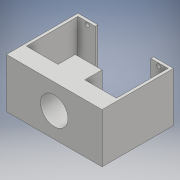
# Autodesk Inventor part: SoporteCuello
Saved by Autodesk Inventor 2017 SP1 (Build 210196100, 196)
## iProperties
Part Number: SoporteCuello
Material: Genérico
Document SubType Name: Modeling
Designer: Juan
Density: 1 g/cm^3
Appearance: Valor por defecto
Author: Juan
Autodesk Inventor part; units mm, degrees
sketch "Boceto1" plane through (0, 0, 0) normal (0, 1, 0) x (-1, 0, 0)
  line L0 (69.5, 36) -> (0, 36)
  line L1 (0, 36) -> (0, 0)
  line L2 (0, 0) -> (69.5, 0)
  line L3 (69.5, 0) -> (69.5, 36)
  dimension "d0" = 69.5
  dimension "d1" = 36
  constraints: 8 end point, 2 parallel, 1 coincident, 1 horizontal, 1 perpendicular
  measures "d0" distance of L2.end L1.end
  measures "d1" distance of L0.end L1.end
extrude "Extrusión1" add sketch "Boceto1" along normal blind 25
ref_plane "Plano de trabajo1" through (0, 25, 0) normal (0, 1, 0) x (1, 0, 0)
sketch "Boceto3" plane through (0, 25, 0) normal (0, 1, 0) x (1, 0, 0)
  line L0 (0, -36) -> (0, 0) projected
  line L1 (-69.5, -36) -> (0, -36) projected
  line L2 (0, 0) -> (-2, 0)
  line L3 (-2, 0) -> (-2, -36)
  line L4 (-2, -36) -> (0, -36)
  line L5 (0, -36) -> (0, 0)
  line L6 (0, 0) -> (-69.5, 0) projected
  line L7 (-69.5, 0) -> (-67.5, 0)
  line L8 (-67.5, 0) -> (-67.5, -36)
  line L9 (-67.5, -36) -> (-69.5, -36)
  line L10 (-69.5, -36) -> (-69.5, 0)
  dimension "d9" = 2
  dimension "d10" = 2
  constraints: 16 end point, 4 parallel, 2 horizontal, 2 perpendicular, 2 point on line
  measures "d9" distance of L4.end L3.end
  measures "d10" distance of L8.end L9.end
extrude "Extrusión3" add sketch "Boceto3" along normal blind 27 contours L1 L3 L2 L0 | L1 L10 L6 L8
ref_plane "Plano de trabajo2" through (-67.5, 25, 36) normal (1, 0, 0) x (0, 0, -1)
ref_plane "Plano de trabajo3" through (-2, 25, 0) normal (-1, 0, 0) x (0, 0, 1)
sketch "Boceto5" plane through (-67.5, 25, 36) normal (1, 0, 0) x (0, 0, -1)
  line L0 (0, 0) -> (0, 27) projected
  line L1 (36, 0) -> (36, 27) projected
  line L2 (0, 27) -> (36, 27)
  line L3 (36, 27) -> (36, 25)
  line L4 (36, 25) -> (0, 25)
  line L5 (0, 25) -> (0, 27)
  point P0 (36, -25)
  dimension "d15" = 2
  constraints: 8 end point, 2 parallel, 1 horizontal, 1 perpendicular, 1 point on line
  measures "d15" distance of L2.end L3.end
sketch "Boceto6" plane through (-2, 25, 0) normal (-1, 0, 0) x (0, 0, 1)
  line L0 (0, 0) -> (0, 27) projected
  line L1 (36, 0) -> (36, 27) projected
  line L2 (0, 27) -> (36, 27)
  line L3 (36, 27) -> (36, 25)
  line L4 (36, 25) -> (0, 25)
  line L5 (0, 25) -> (0, 27)
  point P0 (0, -25)
  dimension "d16" = 2
  constraints: 8 end point, 2 parallel, 1 horizontal, 1 perpendicular, 1 point on line
  measures "d16" distance of L2.end L3.end
extrude "Extrusión4" add sketch "Boceto5" along normal blind 12.5
extrude "Extrusión5" add sketch "Boceto6" along normal blind 12.5
ref_plane "Plano de trabajo4" through (0, 52, 0) normal (0, 1, 0) x (1, 0, 0)
ref_plane "Plano de trabajo5" through (0, 52, 0) normal (0, 1, 0) x (1, 0, 0)
sketch "Boceto7" plane through (0, 52, 0) normal (0, 1, 0) x (1, 0, 0)
  line L0 (0, -36) -> (0, 0) construction
  line L1 (0, -36) -> (-8.75, -36) construction
  line L2 (0, -36) -> (-14.5, -36) construction
  line L3 (-8.75, -36) -> (-8.75, -34) construction
  line L4 (0, 0) -> (-8.75, 0) construction
  line L5 (0, 0) -> (-14.5, 0) construction
  line L6 (-8.75, 0) -> (-8.75, -2) construction
  line L7 (-69.5, -36) -> (0, -36) construction
  line L8 (-69.5, -36) -> (-60.75, -36) construction
  line L9 (-60.75, -36) -> (-60.75, -34) construction
  line L10 (-69.5, 0) -> (-60.75, 0) construction
  line L11 (-60.75, 0) -> (-60.75, -2) construction
  dimension "d23" = 8.75
  dimension "d24" = 2
  dimension "d25" = 8.75
  dimension "d26" = 2
  dimension "d27" = 8.75
  dimension "d28" = 2
  dimension "d29" = 8.75
  constraints: 16 end point, 3 point on line, 2 perpendicular, 2 vertical
  measures "d23" distance of L0.start L1.end
  measures "d24" distance of L1.end L3.end
  measures "d25" distance of L0.end L4.end
  measures "d26" distance of L4.end L6.end
  measures "d27" distance of L7.start L8.end
  measures "d28" distance of L8.end L9.end
  measures "d29" distance of L10.start L10.end
hole "Agujero1" at (-8.75, 52, 34) at (-60.75, 52, 34) at (-60.75, 52, 2) at (-8.75, 52, 2) direction (0, -1, 0) diameter 3 depth 2 tip angle 118
ref_plane "Plano de trabajo6" through (0, 0, 0) normal (0, -1, 0) x (1, 0, 0)
sketch "Boceto8" plane through (0, 0, 0) normal (0, -1, 0) x (1, 0, 0)
  line L0 (0, 36) -> (0, 0) construction
  line L1 (-69.5, 0) -> (-69.5, 36) construction
  line L2 (0, 0) -> (-69.5, 36) construction
  line L3 (-69.5, 0) -> (0, 36) construction
  line L4 (-34.75, 18) -> (-34.75, 36) construction
  line L5 (-69.5, 36) -> (0, 36) construction
  line L6 (-34.75, 18) -> (-16.75, 18) construction
  dimension "d38" = 90
  constraints: 8 end point, 2 midpoint, 1 horizontal, 1 perpendicular
  measures "d38" angle of L6 L4
hole "Agujero2" at (-34.75, 0, 18) direction (0, 1, 0) diameter 20 depth 19 tip angle 118
ref_plane "Plano de trabajo7" through (0, 25, 0) normal (0, 1, 0) x (1, 0, 0)
sketch "Boceto9" plane through (0, 25, 0) normal (0, 1, 0) x (1, 0, 0)
  line L0 (-67.5, -36) -> (-2, -36) projected
  line L1 (-67.5, 0) -> (-44.5, 0)
  line L2 (-44.5, 0) -> (-44.5, -36)
  line L3 (-44.5, -36) -> (-67.5, -36)
  line L4 (-67.5, -36) -> (-67.5, 0)
  line L5 (-2, -36) -> (-2, 0) projected
  line L6 (-2, 0) -> (-25, 0)
  line L7 (-25, 0) -> (-25, -36)
  line L8 (-25, -36) -> (-2, -36)
  line L9 (-2, -36) -> (-2, 0)
  point P0 (0, 0)
  dimension "d47" = 23
  dimension "d48" = 23
  constraints: 16 end point, 4 parallel, 2 horizontal, 2 perpendicular, 2 point on line
  measures "d47" distance of L2.end L3.end
  measures "d48" distance of L8.end L7.end
extrude "Extrusión6" cut sketch "Boceto9" against normal blind 12.5
equation "\"d25\" = d23"
equation "\"d27\" = d23"
equation "\"d29\" = d23"
